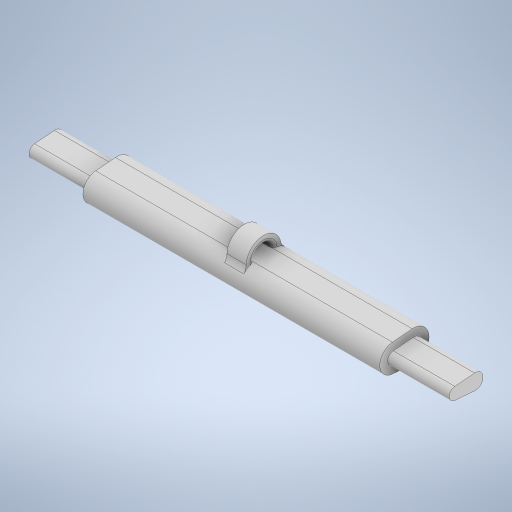
# Autodesk Inventor part: ChargingArm - ConnectingBrace
Saved by Autodesk Inventor 2023 (Build 270158000, 158)
## iProperties
Created: 2023-03-29
Part Number: ChargingArm - ConnectingBrace
Material: Generic
Document SubType Name: Modeling
Designer: Administrator
Density: 1 g/cm^3
Appearance: Default
Author: Administrator
Autodesk Inventor part; units mm, degrees
ref_plane "YZ Plane" through (0, 0, 0) normal (1, 0, 0) x (0, 1, 0)
ref_plane "XZ Plane" through (0, 0, 0) normal (0, 1, 0) x (-1, 0, 0)
ref_plane "XY Plane" through (0, 0, 0) normal (0, 0, 1) x (1, 0, 0)
sketch "Sketch1" plane through (0, 0, 0) normal (1, 0, 0) x (0, 1, 0)
  arc A0 (1.569606, 0.130237) -> (-1.569606, 0.130237) centre (0, 0) ccw
  arc A1 (-1.996639, -5.01633) -> (1.996639, -5.01633) centre (0, -5.182) ccw
  line L0 (1.569606, 0.130237) -> (1.996639, -5.01633)
  line L1 (-1.569606, 0.130237) -> (-1.996639, -5.01633)
  arc A2 (1.996639, -5.01633) -> (-1.996639, -5.01633) centre (0, -5.182) ccw construction
  arc A3 (-1.569606, 0.130237) -> (1.569606, 0.130237) centre (0, 0) ccw construction
  line L2 (3.989789, -4.85095) -> (3.562757, 0.295617)
  arc A4 (3.562757, 0.295617) -> (-3.562757, 0.295617) centre (0, 0) ccw
  line L3 (-3.562757, 0.295617) -> (-3.989789, -4.85095)
  arc A5 (-3.989789, -4.85095) -> (3.989789, -4.85095) centre (0, -5.182) ccw
  arc A6 (3.982998, -4.769105) -> (3.569548, 0.213772) centre (3.776273, -2.277667) ccw
  arc A7 (0.970465, 1.240493) -> (3.672287, -6.776465) centre (3.776273, -2.277667) ccw construction
  arc A8 (2.870948, 2.130325) -> (0.970465, 1.240493) centre (3.776273, -2.277667) ccw construction
  arc A9 (3.672287, -6.776465) -> (2.870948, 2.130325) centre (3.776273, -2.277667) ccw
  arc A10 (1.907157, -3.93791) -> (3.982998, -4.769105) centre (3.776273, -2.277667) ccw construction
  arc A11 (3.569548, 0.213772) -> (1.907157, -3.93791) centre (3.776273, -2.277667) ccw construction
  point P0 (-1.527231, 0.384956)
  point P1 (-1.942735, -4.692312)
  point P2 (1.569795, -0.127934)
  point P3 (1.996879, -5.344741)
  dimension "d12" = 0
  dimension "d0" = 5.182
  dimension "d1" = 0
  dimension "d2" = 3.15
  dimension "d3" = 4.007
  dimension "d4" = 2
  dimension "d9" = 5
  dimension "d10" = 9
  constraints: 31 point on circle, 12 centre point, 8 end point, 4 tangent, 3 point on line, 2 coincident, 1 midpoint, 3 other
  measures "d0" distance of A0.centre A1.centre
  measures "d1" horizontal distance of A0.centre A1.centre
  measures "d2" diameter of A0
  measures "d3" diameter of A1
  measures "d4" radial gap between concentric circles of A1 A5
  measures "d9" diameter of A6
  measures "d10" diameter of A7
extrude "Extrusion1" add sketch "Sketch1" along normal mid plane 77 contours L0 A1 L1 A0 | A5 L3 A4 L2
extrude "Extrusion2" add sketch "Sketch1" along normal mid plane 109 contours L0 A1 L1 A0
extrude "Extrusion3" add sketch "Sketch1" along normal mid plane 5 contours L2 A6 A4 A9 A5
fillet "Fillet1" radius 3 2 edges at (0, 3.6723, -6.7765) (0, 2.8709, 2.1303)
fillet "Fillet2" radius 1 2 edges at (2.5, 6.2677, -2.0709) (-2.5, 6.2677, -2.0709)
body "Solid1"
